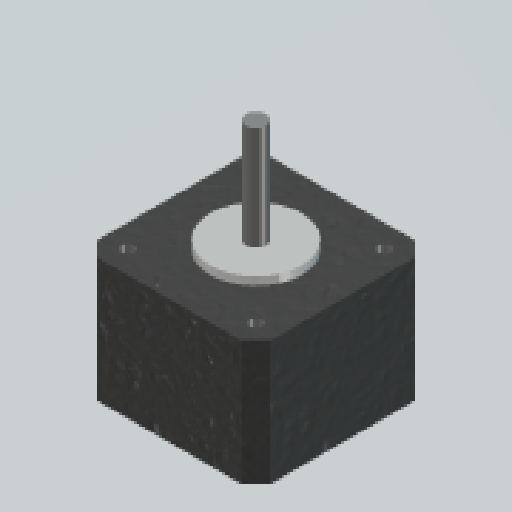
# Autodesk Inventor part: Extruder Motor
Saved by Autodesk Inventor 2023.2 (Build 272271000, 271)
## iProperties
Created: 2020-05-09
Part Number: Extruder Motor
Material: Steel, Alloy
Document SubType Name: Modeling
Designer: Remo
Mass: 814.637 g
Surface Area: 139.042 cm^2
Volume: 105.386 cm^3
Density: 7.73 g/cm^3
Appearance: Semi-Polished
Description: E3D - Super Whopper Motor
Author: Remo
Autodesk Inventor part; units mm, degrees
ref_plane "YZ Plane" through (0, 0, 0) normal (1, 0, 0) x (0, 1, 0)
ref_plane "XZ Plane" through (0, 0, 0) normal (0, 1, 0) x (-1, 0, 0)
ref_plane "XY Plane" through (0, 0, 0) normal (0, 0, 1) x (1, 0, 0)
sketch "Sketch1" plane through (0, 0, 0) normal (0, 0, 1) x (1, 0, 0)
  line L0 (21, -21) -> (-21, -21)
  line L1 (-21, -21) -> (-21, 21)
  line L2 (-21, 21) -> (21, 21)
  line L3 (21, 21) -> (21, -21)
  line L4 (21, -21) -> (-21, 21) construction
  line L5 (-21, -21) -> (21, 21) construction
  point P0 (0, 0)
  dimension "d0" = 42
  constraints: 12 end point, 2 midpoint, 2 parallel, 2 perpendicular, 1 horizontal
  measures "d0" distance of L1.end L2.end
extrude "Extrusion1" add sketch "Sketch1" along normal blind 30
sketch "Sketch2" plane through (0, 0, 30) normal (0, 0, 1) x (1, 0, 0)
  point P0 (0, 0)
  point P1 (-15.5, 15.5)
  point P2 (-15.5, -15.5)
  point P3 (15.5, -15.5)
  point P4 (15.5, 15.5)
  dimension "d3" = 31
  dimension "d4" = 31
  dimension "d5" = 15.5
  dimension "d6" = 15.5
  constraints: 2 horizontal alignment, 2 vertical alignment
  measures "d3" distance of point (-15.5, 15.5) point (15.5, 15.5)
  measures "d4" distance of point (-15.5, -15.5) point (-15.5, 15.5)
  measures "d5" horizontal distance of point (-15.5, 15.5) point (0, 0)
  measures "d6" horizontal distance of point (-15.5, 15.5) point (0, 0)
hole "Hole1" at (-15.5, 15.5, 30) at (-15.5, -15.5, 30) at (15.5, -15.5, 30) at (15.5, 15.5, 30) direction (0, 0, -1) diameter 3 depth 8 tip angle 118
chamfer "Chamfer1" distance 3.5 angle 45 4 edges at (21, 21, 15) (21, -21, 15) (-21, 21, 15) (-21, -21, 15)
sketch "Sketch3" plane through (0, 0, 30) normal (0, 0, 1) x (1, 0, 0)
  circle A0 centre (0, 0) radius 11
  dimension "d17" = 22
  constraints: 1 centre point, 1 coincident
  measures "d17" diameter of A0
extrude "Extrusion2" add sketch "Sketch3" along normal blind 2
sketch "Sketch4" plane through (0, 0, 32) normal (0, 0, 1) x (1, 0, 0)
  circle A0 centre (0, 0) radius 11 projected
  circle A1 centre (0, 0) radius 2.5
  dimension "d20" = 5
  constraints: 1 centre point, 1 coincident
  measures "d20" diameter of A1
extrude "Extrusion3" add sketch "Sketch4" along normal blind 25 contours A1
equation "\"d4\" = d3"
equation "\"d5\" = 0.5 * d3"
equation "\"d6\" = 0.5 * d3"
body "Solid1"
